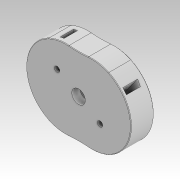
# Autodesk Inventor part: Rotor_NEW
Saved by Autodesk Inventor 2020 (Build 240168000, 168)
## iProperties
Created: 2022-01-30
Part Number: Rotor_NEW
Material: Generic
Document SubType Name: Modeling
Designer: DDeGo
Density: 1 g/cm^3
Appearance: Default
Author: DDeGo
Autodesk Inventor part; units mm, degrees
ref_plane "YZ Plane" through (0, 0, 0) normal (1, 0, 0) x (0, 1, 0)
ref_plane "XZ Plane" through (0, 0, 0) normal (0, 1, 0) x (-1, 0, 0)
ref_plane "XY Plane" through (0, 0, 0) normal (0, 0, 1) x (1, 0, 0)
sketch "Sketch1" plane through (0, 0, 0) normal (0, 0, 1) x (1, 0, 0)
  line L0 (4.8, 0) -> (-4.8, 0) construction
  line L1 (4.8, 14.7) -> (-4.8, 14.7) construction
  arc A0 (19.5, 0) -> (11.1318, 13.2664) centre (4.8, 0) ccw
  arc A1 (-4.8, 14.7) -> (-11.1318, 13.2664) centre (-4.8, 0) ccw construction
  line L2 (-19.5, 24.8831) -> (19.5, 24.8831) construction
  line L3 (19.5, 24.8831) -> (19.5, -24.8831) construction
  line L4 (19.5, -24.8831) -> (-19.5, -24.8831) construction
  line L5 (-19.5, -24.8831) -> (-19.5, 24.8831) construction
  line L6 (0, 0) -> (0, 14.7) construction
  arc A2 (-3.6434, 14.6131) -> (0, 14.45) centre (0, 55.2356) ccw
  arc A3 (-3.6434, 14.6131) -> (-11.1318, 13.2664) centre (-4.9297, 0.2718) ccw
  arc A4 (-11.1318, 13.2664) -> (-19.5, 0) centre (-4.8, 0) ccw
  arc A5 (0, 14.45) -> (3.6434, 14.6131) centre (0, 55.2356) ccw
  arc A6 (11.1318, 13.2664) -> (3.6434, 14.6131) centre (4.9297, 0.2718) ccw
  arc A7 (11.1318, 13.2664) -> (4.8, 14.7) centre (4.8, 0) ccw construction
  line L7 (-19.5, 0) -> (19.5, 0) construction
  arc A8 (11.1318, -13.2664) -> (19.5, 0) centre (4.8, 0) ccw
  arc A9 (0, -14.45) -> (-3.6434, -14.6131) centre (0, -55.2356) ccw
  arc A10 (-11.1318, -13.2664) -> (-3.6434, -14.6131) centre (-4.9297, -0.2718) ccw
  arc A11 (-19.5, 0) -> (-11.1318, -13.2664) centre (-4.8, 0) ccw
  arc A12 (3.6434, -14.6131) -> (0, -14.45) centre (0, -55.2356) ccw
  arc A13 (3.6434, -14.6131) -> (11.1318, -13.2664) centre (4.9297, -0.2718) ccw
  circle A14 centre (0, 0) radius 2.5
  line L8 (-11.1318, 13.2664) -> (0, 0) construction
  line L9 (-3.6434, 14.6131) -> (0, 0) construction
  dimension "d0" = 14.7
  dimension "d1" = 39
  dimension "d2" = 0.25
  dimension "d5" = 5
  dimension "d14" = 40
  dimension "d15" = 14
  constraints: 28 point on circle, 22 end point, 15 centre point, 12 tangent, 9 symmetric about line, 5 midpoint, 3 point on line, 2 equal radius, 2 horizontal, 2 parallel, 1 coincident, 1 perpendicular, 1 vertical, 6 other
  measures "d0" radius of A1
  measures "d1" distance of L2.start L2.end
  measures "d2" distance from line of L1 A2.end
  measures "d5" diameter of A14
  measures "d14" angle of L6 L8
  measures "d15" angle of L6 L9
extrude "Extrusion1" add sketch "Sketch1" along normal mid plane 8 contours A8 A13 A12 A9 A10 A11 A4 A3 A2 A5 A6 A0 | A14
sketch "Sketch2" plane through (0, 0, 0) normal (0, 1, 0) x (-1, 0, 0)
  line L0 (0, 0) -> (0, 4) construction
  line L1 (0, 4) -> (2.52, 4)
  line L2 (-3.6434, 4) -> (3.6434, 4) construction
  line L3 (3.6434, 4) -> (11.1318, 4) construction
  line L4 (11.1318, 4) -> (11.1318, 4) construction
  line L5 (11.1318, 4) -> (3.6434, 4) construction
  line L6 (3.6434, 4) -> (-3.6434, 4) construction
  line L7 (-3.6434, 4) -> (-11.1318, 4) construction
  line L8 (-11.1318, 4) -> (-11.1318, 4) construction
  line L9 (-11.1318, 4) -> (-3.6434, 4) construction
  line L10 (2.52, -4) -> (0, -4)
  line L11 (0, -4) -> (0, 4)
  line L12 (3.6434, -4) -> (-3.6434, -4) projected
  line L13 (-3.6434, -4) -> (-11.1318, -4) projected
  line L14 (-11.1318, -4) -> (-11.1318, -4) projected
  line L15 (-11.1318, -4) -> (-3.6434, -4) projected
  line L16 (-3.6434, -4) -> (3.6434, -4) projected
  line L17 (3.6434, -4) -> (11.1318, -4) projected
  line L18 (11.1318, -4) -> (11.1318, -4) projected
  line L19 (11.1318, -4) -> (3.6434, -4) projected
  line L20 (2.52, -1) -> (2.02, -0.7113)
  line L21 (2.02, -0.7113) -> (2.02, 0.7113)
  line L22 (2.02, 0.7113) -> (2.52, 1)
  line L23 (2.52, 4) -> (2.52, 1)
  line L24 (2.52, -1) -> (2.52, -4)
  dimension "d53" = 2.52
  dimension "d54" = 0.5
  dimension "d55" = 60
  dimension "d56" = 3
  dimension "d57" = 3
  constraints: 18 end point, 2 collinear, 2 midpoint, 2 perpendicular, 2 vertical, 1 equal length, 1 horizontal, 1 point on line
  measures "d53" distance between parallel lines of L24 L11
  measures "d54" distance between parallel lines of L24 L21
  measures "d55" angle of L24 L20
  measures "d56" distance of L1.end L22.end
  measures "d57" distance of L20.start L10.start
revolve "Revolution1" cut sketch "Sketch2" angle 360 about axis through (0, 0, 0) along (0, 0, 1)
sketch "Sketch3" plane through (0, 0, -4) normal (0, 0, -1) x (-1, 0, 0)
  circle A0 centre (0, 0) radius 12.5
  circle A1 centre (0, 0) radius 2.5 projected
  dimension "d18" = 25
  constraints: 1 centre point, 1 coincident
  measures "d18" diameter of A0
extrude "Extrusion2" add sketch "Sketch3" along normal blind 10
spur gear teeth "Spur Gear1" teeth 16 pitch diameter 9.6 tip diameter 10.6669 root diameter 7.9669 face width 3 trims to tip circle yes start plane through (0, 0, -14) normal (0, 0, -1) x (-1, 0, 0)
ref_plane "Work Plane1" through (0, 0, -0.5) normal (0, 0, -1) x (-1, 0, 0)
sketch "Sketch4" plane through (0, 0, -11) normal (0, 0, -1) x (-1, 0, 0)
  arc A0 (3.9518, 3.5817) -> (3.5817, 3.9518) centre (0, 0) ccw projected
  arc A1 (3.1996, 2.3729) -> (3.9518, 3.5817) centre (-0.1257, 5.2809) ccw projected
  arc A2 (4.8214, 2.2804) -> (3.4167, 2.0479) centre (4.8308, -2.137) ccw projected
  arc A3 (5.0217, 1.7968) -> (4.8214, 2.2804) centre (0, 0) ccw projected
  arc A4 (3.8641, 0.9679) -> (5.0217, 1.7968) centre (1.9048, 4.927) ccw projected
  arc A5 (5.327, 0.2617) -> (3.9404, 0.5845) centre (3.6453, -3.823) ccw projected
  arc A6 (5.327, -0.2617) -> (5.327, 0.2617) centre (0, 0) ccw projected
  arc A7 (3.9404, -0.5845) -> (5.327, -0.2617) centre (3.6453, 3.823) ccw projected
  arc A8 (5.0217, -1.7968) -> (3.8641, -0.9679) centre (1.9048, -4.927) ccw projected
  arc A9 (4.8214, -2.2804) -> (5.0217, -1.7968) centre (0, 0) ccw projected
  arc A10 (3.4167, -2.0479) -> (4.8214, -2.2804) centre (4.8308, 2.137) ccw projected
  arc A11 (3.9518, -3.5817) -> (3.1996, -2.3729) centre (-0.1257, -5.2809) ccw projected
  arc A12 (3.5817, -3.9518) -> (3.9518, -3.5817) centre (0, 0) ccw projected
  arc A13 (2.3729, -3.1996) -> (3.5817, -3.9518) centre (5.2809, 0.1257) ccw projected
  arc A14 (2.2804, -4.8214) -> (2.0479, -3.4167) centre (-2.137, -4.8308) ccw projected
  arc A15 (1.7968, -5.0217) -> (2.2804, -4.8214) centre (0, 0) ccw projected
  arc A16 (0.9679, -3.8641) -> (1.7968, -5.0217) centre (4.927, -1.9048) ccw projected
  arc A17 (0.2617, -5.327) -> (0.5845, -3.9404) centre (-3.823, -3.6453) ccw projected
  arc A18 (-0.2617, -5.327) -> (0.2617, -5.327) centre (0, 0) ccw projected
  arc A19 (-0.5845, -3.9404) -> (-0.2617, -5.327) centre (3.823, -3.6453) ccw projected
  arc A20 (-1.7968, -5.0217) -> (-0.9679, -3.8641) centre (-4.927, -1.9048) ccw projected
  arc A21 (-2.2804, -4.8214) -> (-1.7968, -5.0217) centre (0, 0) ccw projected
  arc A22 (-2.0479, -3.4167) -> (-2.2804, -4.8214) centre (2.137, -4.8308) ccw projected
  arc A23 (-3.5817, -3.9518) -> (-2.3729, -3.1996) centre (-5.2809, 0.1257) ccw projected
  arc A24 (-3.9518, -3.5817) -> (-3.5817, -3.9518) centre (0, 0) ccw projected
  arc A25 (-3.1996, -2.3729) -> (-3.9518, -3.5817) centre (0.1257, -5.2809) ccw projected
  arc A26 (-4.8214, -2.2804) -> (-3.4167, -2.0479) centre (-4.8308, 2.137) ccw projected
  arc A27 (-5.0217, -1.7968) -> (-4.8214, -2.2804) centre (0, 0) ccw projected
  arc A28 (-3.8641, -0.9679) -> (-5.0217, -1.7968) centre (-1.9048, -4.927) ccw projected
  arc A29 (-5.327, -0.2617) -> (-3.9404, -0.5845) centre (-3.6453, 3.823) ccw projected
  arc A30 (-5.327, 0.2617) -> (-5.327, -0.2617) centre (0, 0) ccw projected
  arc A31 (-3.9404, 0.5845) -> (-5.327, 0.2617) centre (-3.6453, -3.823) ccw projected
  arc A32 (-5.0217, 1.7968) -> (-3.8641, 0.9679) centre (-1.9048, 4.927) ccw projected
  arc A33 (-4.8214, 2.2804) -> (-5.0217, 1.7968) centre (0, 0) ccw projected
  arc A34 (-3.4167, 2.0479) -> (-4.8214, 2.2804) centre (-4.8308, -2.137) ccw projected
  arc A35 (-3.9518, 3.5817) -> (-3.1996, 2.3729) centre (0.1257, 5.2809) ccw projected
  arc A36 (-3.5817, 3.9518) -> (-3.9518, 3.5817) centre (0, 0) ccw projected
  arc A37 (-2.3729, 3.1996) -> (-3.5817, 3.9518) centre (-5.2809, -0.1257) ccw projected
  arc A38 (-2.2804, 4.8214) -> (-2.0479, 3.4167) centre (2.137, 4.8308) ccw projected
  arc A39 (-1.7968, 5.0217) -> (-2.2804, 4.8214) centre (0, 0) ccw projected
  arc A40 (-0.9679, 3.8641) -> (-1.7968, 5.0217) centre (-4.927, 1.9048) ccw projected
  arc A41 (-0.2617, 5.327) -> (-0.5845, 3.9404) centre (3.823, 3.6453) ccw projected
  arc A42 (0.2617, 5.327) -> (-0.2617, 5.327) centre (0, 0) ccw projected
  arc A43 (0.5845, 3.9404) -> (0.2617, 5.327) centre (-3.823, 3.6453) ccw projected
  arc A44 (1.7968, 5.0217) -> (0.9679, 3.8641) centre (4.927, 1.9048) ccw projected
  arc A45 (2.2804, 4.8214) -> (1.7968, 5.0217) centre (0, 0) ccw projected
  arc A46 (2.0479, 3.4167) -> (2.2804, 4.8214) centre (-2.137, 4.8308) ccw projected
  arc A47 (3.5817, 3.9518) -> (2.3729, 3.1996) centre (5.2809, -0.1257) ccw projected
  circle A48 centre (0, 0) radius 12.5 projected
  arc A49 (3.4167, 2.0479) -> (3.1996, 2.3729) centre (0, 0) ccw projected
  arc A50 (3.9404, 0.5845) -> (3.8641, 0.9679) centre (0, 0) ccw projected
  arc A51 (3.8641, -0.9679) -> (3.9404, -0.5845) centre (0, 0) ccw projected
  arc A52 (3.1996, -2.3729) -> (3.4167, -2.0479) centre (0, 0) ccw projected
  arc A53 (2.0479, -3.4167) -> (2.3729, -3.1996) centre (0, 0) ccw projected
  arc A54 (0.5845, -3.9404) -> (0.9679, -3.8641) centre (0, 0) ccw projected
  arc A55 (-0.9679, -3.8641) -> (-0.5845, -3.9404) centre (0, 0) ccw projected
  arc A56 (-2.3729, -3.1996) -> (-2.0479, -3.4167) centre (0, 0) ccw projected
  arc A57 (-3.4167, -2.0479) -> (-3.1996, -2.3729) centre (0, 0) ccw projected
  arc A58 (-3.9404, -0.5845) -> (-3.8641, -0.9679) centre (0, 0) ccw projected
  arc A59 (-3.8641, 0.9679) -> (-3.9404, 0.5845) centre (0, 0) ccw projected
  arc A60 (-3.1996, 2.3729) -> (-3.4167, 2.0479) centre (0, 0) ccw projected
  arc A61 (-2.0479, 3.4167) -> (-2.3729, 3.1996) centre (0, 0) ccw projected
  arc A62 (-0.5845, 3.9404) -> (-0.9679, 3.8641) centre (0, 0) ccw projected
  arc A63 (0.9679, 3.8641) -> (0.5845, 3.9404) centre (0, 0) ccw projected
  arc A64 (2.3729, 3.1996) -> (2.0479, 3.4167) centre (0, 0) ccw projected
  point P0 (0, 0)
extrude "Extrusion3" cut sketch "Sketch4" against normal up to surface (10.5 mm away)
ref_plane "Work Plane2" through (0, 0, -3.75) normal (0, 0, -1) x (-1, 0, 0)
sketch "Sketch5" plane through (0, 0, -14) normal (0, 0, -1) x (-1, 0, 0)
  circle A0 centre (0, 0) radius 7.9397
  constraints: 1 centre point, 1 coincident
extrude "Extrusion4" cut sketch "Sketch5" against normal up to surface (10.25 mm away)
fillet "Fillet1" radius 0.3 32 edges at (-1.7968, -5.0217, -2.125) (-2.2804, -4.8214, -2.125) (-3.5817, -3.9518, -2.125) (-3.9518, -3.5817, -2.125) (-5.0217, -1.7968, -2.125) (-4.8214, -2.2804, -2.125) (-5.327, -0.2617, -2.125) (-5.327, 0.2617, -2.125) (-5.0217, 1.7968, -2.125) (-4.8214, 2.2804, -2.125) (-3.9518, 3.5817, -2.125) (-3.5817, 3.9518, -2.125) (-2.2804, 4.8214, -2.125) (-1.7968, 5.0217, -2.125) (-0.2617, 5.327, -2.125) (0.2617, 5.327, -2.125) (2.2804, 4.8214, -2.125) (1.7968, 5.0217, -2.125) (3.5817, 3.9518, -2.125) (3.9518, 3.5817, -2.125) (4.8214, 2.2804, -2.125) (5.0217, 1.7968, -2.125) (5.327, 0.2617, -2.125) (5.327, -0.2617, -2.125) (5.0217, -1.7968, -2.125) (4.8214, -2.2804, -2.125) (3.9518, -3.5817, -2.125) (3.5817, -3.9518, -2.125) (2.2804, -4.8214, -2.125) (1.7968, -5.0217, -2.125) (0.2617, -5.327, -2.125) (-0.2617, -5.327, -2.125)
fillet "Fillet2" radius 1 1 edges at (12.5, 0, -0.5)
sketch "Sketch6" plane through (0, 0, 4) normal (0, 0, 1) x (1, 0, 0)
  circle A0 centre (8, -4.8) radius 1
  circle A1 centre (9.6805, -3.2071) radius 1.1297 construction
  line L0 (0, 0) -> (8, -4.8) construction
  line L1 (8, -4.8) -> (8, 0) construction
  line L2 (8, 0) -> (0, 0) construction
  dimension "d28" = 8
  dimension "d29" = 4.8
  dimension "d30" = 2
  constraints: 6 end point, 2 centre point, 1 perpendicular, 1 vertical
  measures "d28" distance of L1.end L0.start
  measures "d29" distance of L0.end L1.end
  measures "d30" diameter of A0
extrude "Extrusion5" cut sketch "Sketch6" against normal blind 3.5
sketch "Sketch7" plane through (8, -4.8, 0.5) normal (0, 0, 1) x (1, 0, 0)
  circle A0 centre (0, 0) radius 1 construction
  line L0 (0, 0) -> (10.4256, 18.0576) construction
  line L1 (-0.866, 0.5) -> (9.5595, 18.5576)
  line L2 (11.2916, 17.5576) -> (0.866, -0.5)
  arc A1 (-0.866, 0.5) -> (0.866, -0.5) centre (0, 0) ccw
  arc A2 (11.2916, 17.5576) -> (9.5595, 18.5576) centre (10.4256, 18.0576) ccw
  circle A3 centre (0, 0) radius 1 projected
  line L3 (0, 0) -> (0, 4.6154) construction
  point P0 (-8, 4.8)
  point P1 (5.2128, 9.0288)
  point P2 (-0.866, 0.5)
  point P3 (0.866, -0.5)
  dimension "d33" = 30
  constraints: 10 end point, 4 point on circle, 4 tangent, 2 centre point, 1 concentric, 1 midpoint, 1 parallel, 1 vertical
  measures "d33" angle of L0 L3
extrude "Extrusion6" cut sketch "Sketch7" along normal blind 2.5 contours L1 A2 L2 A3
sketch "Sketch8" plane through (15.4603, 10.1216, 3) normal (0.8660254, -0.5, 0) x (0, 0, -1)
  line L0 (0, 0) -> (2.5, 0) construction
  line L1 (0, 0) -> (0, -16.6527) construction
  line L2 (2.5, -16.6527) -> (0, -16.6527) construction
  line L3 (2.5, 0) -> (2.5, -16.6527) construction
  line L4 (2.5, 0) -> (2.5, -16.6527) construction
  line L5 (2.5, -7.6527) -> (5.5, 0)
  line L6 (5.5, 0) -> (2.5, 0)
  line L7 (7, 0.5592) -> (-1, 0.5592) construction
  line L8 (2.5, 0) -> (2.5, -7.6527)
  line L9 (7, -22.4189) -> (7, 0.6042) construction
  point P0 (3, -16.4958)
  dimension "d36" = 9
  dimension "d38" = 1.5
  constraints: 6 end point, 1 parallel, 1 perpendicular, 1 point on line
  measures "d36" distance from line of L5.start L2
  measures "d38" distance from line of L9 L5.end
extrude "Extrusion7" cut sketch "Sketch8" along normal up to surface (2 mm away)
sketch "Sketch9" plane through (0, 0, 0) normal (0, 0, 1) x (1, 0, 0)
  line L0 (7.1255, -15.5449) -> (6.7355, -13.5833)
  line L1 (6.7355, -13.5833) -> (8.2068, -13.2908)
  line L2 (8.2068, -13.2908) -> (8.5967, -15.2525)
  line L3 (8.5967, -15.2525) -> (7.1255, -15.5449)
  line L4 (7.1255, -15.5449) -> (8.2068, -13.2908) construction
  line L5 (6.7355, -13.5833) -> (8.5967, -15.2525) construction
  arc A0 (11.1318, -13.2664) -> (11.1318, 13.2664) centre (4.8, 0) ccw projected
  arc A1 (3.6434, -14.6131) -> (11.1318, -13.2664) centre (4.9297, -0.2718) ccw projected
  line L6 (7.6661, -14.4179) -> (7.4711, -13.4371)
  line L7 (0, 0) -> (7.6661, -14.4179) construction
  circle A2 centre (0, 0) radius 2.02 projected
  line L8 (0, 0) -> (0, -15.7126) construction
  dimension "d43" = 1.5
  dimension "d44" = 2
  dimension "d58" = 28
  constraints: 18 end point, 4 midpoint, 2 parallel, 1 line through centre, 1 perpendicular, 1 point on circle, 1 vertical
  measures "d43" distance between parallel lines of L0 L2
  measures "d44" distance between parallel lines of L3 L1
  measures "d58" angle of L7 L8
extrude "Extrusion8" cut sketch "Sketch9" against normal mid plane 5 contours L0 A1 L2 L3 | L0 L1 L6 A1 | L6 L1 L2 A1
sketch "Sketch10" plane through (8.3798, -14.1615, -2.5) normal (-0.9808083, -0.1949744, 0) x (0, 0, 1)
  line L0 (5, -0.0871) -> (5, 0.8877) projected
  line L1 (0, 0.8877) -> (5, 0.8877) projected
  line L2 (0, 0.8877) -> (0, -0.0871) projected
  line L3 (0, 0.8877) -> (5, 0.8877) projected
  line L4 (5, 0.8877) -> (1, 7.0236)
  line L5 (1, 7.0236) -> (-1.5, 7.0236)
  line L6 (-1.5, 7.0236) -> (0, 0.8877)
  line L7 (-1.5, 3.0236) -> (-1.5, 28.0236) construction
  line L8 (-1.5, 30.5666) -> (-1.5, 29.1458) projected
  line L9 (-1.5, 29.1458) -> (-1.5, 26.365) projected
  line L10 (-1.5, 26.365) -> (-1.5, 0.3414) construction
  line L11 (-1.5, 0.3414) -> (-1.5, 0.4806) construction
  line L12 (-1.5, 0.4806) -> (-1.5, 1.9014) construction
  line L13 (-1.5, 1.9014) -> (-1.5, 4.6822) construction
  line L14 (-1.5, 4.6822) -> (-1.5, 30.7058) construction
  line L15 (-1.5, 30.7058) -> (-1.5, 30.5666) projected
  line L16 (-1.5, 3.0236) -> (-1.5, 28.0236) construction
  line L17 (1, 28.0236) -> (1, 3.0236) construction
  line L18 (-1.5, 3.0236) -> (1, 3.0236) construction
  line L19 (5, -0.0871) -> (0, -0.0871) projected
  point P0 (2.5, 15.5236)
  dimension "d45" = 4
  constraints: 6 end point, 2 point on line, 1 parallel
  measures "d45" distance from line of L18 L5.end
extrude "Extrusion9" cut sketch "Sketch10" along normal up to surface (1.5 mm away) contours L1 L6 L5 L4
fillet "Fillet3" radius 2 6 edges at (6.1937, -10.8576, -2.3397) (5.9127, -9.4441, -0.5) (6.1323, -10.5485, -0.7873) (7.3181, -8.8206, -0.5) (7.5457, -9.9655, -2.4144) (7.4795, -9.6324, -0.7813)
pattern_circular "Circular Pattern1" count 2 over 360 about axis through (0, 0, -2.5) along (0, 0, -1) of "Extrusion5", "Extrusion6", "Extrusion7", "Extrusion8", "Extrusion9", "Fillet3"
sketch "Sketch12" plane through (0, 0, -4) normal (0, 0, -1) x (-1, 0, 0)
  circle A0 centre (0, 0) radius 12.5 projected
  arc A1 (-3.6434, 14.6131) -> (3.6434, 14.6131) centre (0, 55.2356) ccw projected
  arc A2 (-3.6434, 14.6131) -> (-11.1318, 13.2664) centre (-4.9297, 0.2718) ccw projected
  arc A3 (-11.1318, 13.2664) -> (-11.1318, -13.2664) centre (-4.8, 0) ccw projected
  arc A4 (-11.1318, -13.2664) -> (-3.6434, -14.6131) centre (-4.9297, -0.2718) ccw projected
  arc A5 (3.6434, -14.6131) -> (-3.6434, -14.6131) centre (0, -55.2356) ccw projected
  arc A6 (3.6434, -14.6131) -> (11.1318, -13.2664) centre (4.9297, -0.2718) ccw projected
  arc A7 (11.1318, -13.2664) -> (11.1318, 13.2664) centre (4.8, 0) ccw projected
  arc A8 (11.1318, 13.2664) -> (3.6434, 14.6131) centre (4.9297, 0.2718) ccw projected
  arc A9 (3.7328, -13.6171) -> (10.7011, -12.3639) centre (4.9297, -0.2718) ccw
  arc A10 (3.7328, -13.6171) -> (-3.7328, -13.6171) centre (0, -55.2356) ccw
  arc A11 (-10.7011, -12.3639) -> (-3.7328, -13.6171) centre (-4.9297, -0.2718) ccw
  arc A12 (-10.7011, 12.3639) -> (-10.7011, -12.3639) centre (-4.8, 0) ccw
  arc A13 (-3.7328, 13.6171) -> (-10.7011, 12.3639) centre (-4.9297, 0.2718) ccw
  arc A14 (-3.7328, 13.6171) -> (3.7328, 13.6171) centre (0, 55.2356) ccw
  arc A15 (10.7011, 12.3639) -> (3.7328, 13.6171) centre (4.9297, 0.2718) ccw
  arc A16 (10.7011, -12.3639) -> (10.7011, 12.3639) centre (4.8, 0) ccw
  dimension "d0" = 14.7
  dimension "d1" = 39
  dimension "d2" = 0.25
  dimension "d5" = 5
  dimension "d14" = 40
  dimension "d15" = 14
  dimension "d60" = 1
  constraints: 16 point on circle, 8 centre point, 7 other
  measures "d60" radial gap between concentric circles of A6 A9
extrude "Extrusion10" add sketch "Sketch12" along normal blind 0.5 contours A1 A8 A7 A6 A5 A4 A3 A2
fillet "Fillet4" radius 10 1 edges at (12.5, 2.9942, 0.5)
sketch "Sketch13" plane through (3.823, -3.6453, -3.75) normal (0, 0, -1) x (-0.9789933, -0.2038926, 0)
  arc A0 (4.1422, -0.8614) -> (4.3751, -0.6098) centre (4.0779, -0.5684) ccw projected
  arc A1 (4.3751, -0.6098) -> (4.3751, 0.6098) centre (0, 0) ccw projected
  arc A2 (4.3751, 0.6098) -> (4.7349, 0.7626) centre (2.9994, 4.3482) ccw projected
  arc A3 (4.7349, 0.7626) -> (5.6126, -0.0841) centre (8.2113, 3.488) ccw projected
  arc A4 (5.6126, -0.0841) -> (5.9554, -0.0912) centre (5.7891, 0.1585) ccw projected
  arc A5 (5.9554, -0.0912) -> (6.0489, -0.0275) centre (2.9994, 4.3482) ccw projected
  arc A6 (6.0489, -0.0275) -> (6.1677, 0.294) centre (5.8773, 0.2186) ccw projected
  arc A7 (6.1677, 0.294) -> (5.701, 1.4208) centre (1.8923, -0.8169) ccw projected
  arc A8 (5.701, 1.4208) -> (5.9749, 1.6997) centre (2.9994, 4.3482) ccw projected
  arc A9 (5.9749, 1.6997) -> (7.1099, 1.2533) centre (8.1438, 5.5479) ccw projected
  arc A10 (7.1099, 1.2533) -> (7.4292, 1.3779) centre (7.1801, 1.545) ccw projected
  arc A11 (7.4292, 1.3779) -> (7.4913, 1.4725) centre (2.9994, 4.3482) ccw projected
  arc A12 (7.4913, 1.4725) -> (7.478, 1.8151) centre (7.2386, 1.6343) ccw projected
  arc A13 (7.478, 1.8151) -> (6.6156, 2.6775) centre (3.9532, -0.8474) ccw projected
  arc A14 (6.6156, 2.6775) -> (6.762, 3.0399) centre (2.9994, 4.3482) ccw projected
  arc A15 (6.762, 3.0399) -> (7.9813, 3.0619) centre (7.2931, 7.4253) ccw projected
  arc A16 (7.9813, 3.0619) -> (8.2287, 3.2992) centre (7.9346, 3.3582) ccw projected
  arc A17 (8.2287, 3.2992) -> (8.2498, 3.4104) centre (2.9994, 4.3482) ccw projected
  arc A18 (8.2498, 3.4104) -> (8.1065, 3.7218) centre (7.9545, 3.4631) ccw projected
  arc A19 (8.1065, 3.7218) -> (6.9797, 4.1885) centre (5.8688, -0.0869) ccw projected
  arc A20 (6.9797, 4.1885) -> (6.9762, 4.5794) centre (2.9994, 4.3482) ccw projected
  arc A21 (6.9762, 4.5794) -> (8.0944, 5.0663) centre (5.7887, 8.8341) ccw projected
  arc A22 (8.0944, 5.0663) -> (8.2321, 5.3802) centre (7.9378, 5.3222) ccw projected
  arc A23 (8.2321, 5.3802) -> (8.209, 5.491) centre (2.9994, 4.3482) ccw projected
  arc A24 (8.209, 5.491) -> (7.9574, 5.7238) centre (7.916, 5.4267) ccw projected
  arc A25 (7.9574, 5.7238) -> (6.7378, 5.7238) centre (7.3476, 1.3487) ccw projected
  arc A26 (6.7378, 5.7238) -> (6.585, 6.0836) centre (2.9994, 4.3482) ccw projected
  arc A27 (6.585, 6.0836) -> (7.4318, 6.9613) centre (3.8597, 9.5601) ccw projected
  arc A28 (7.4318, 6.9613) -> (7.4389, 7.3041) centre (7.1892, 7.1378) ccw projected
  arc A29 (7.4389, 7.3041) -> (7.3752, 7.3976) centre (2.9994, 4.3482) ccw projected
  arc A30 (7.3752, 7.3976) -> (7.0536, 7.5164) centre (7.129, 7.2261) ccw projected
  arc A31 (7.0536, 7.5164) -> (5.9269, 7.0497) centre (8.1645, 3.241) ccw projected
  arc A32 (5.9269, 7.0497) -> (5.648, 7.3237) centre (2.9994, 4.3482) ccw projected
  arc A33 (5.648, 7.3237) -> (6.0944, 8.4586) centre (1.7997, 9.4925) ccw projected
  arc A34 (6.0944, 8.4586) -> (5.9698, 8.778) centre (5.8027, 8.5288) ccw projected
  arc A35 (5.9698, 8.778) -> (5.8751, 8.84) centre (2.9994, 4.3482) ccw projected
  arc A36 (5.8751, 8.84) -> (5.5326, 8.8267) centre (5.7134, 8.5873) ccw projected
  arc A37 (5.5326, 8.8267) -> (4.6702, 7.9644) centre (8.195, 5.3019) ccw projected
  arc A38 (4.6702, 7.9644) -> (4.3077, 8.1107) centre (2.9994, 4.3482) ccw projected
  arc A39 (4.3077, 8.1107) -> (4.2858, 9.3301) centre (-0.0776, 8.6418) ccw projected
  arc A40 (4.2858, 9.3301) -> (4.0484, 9.5775) centre (3.9894, 9.2833) ccw projected
  arc A41 (4.0484, 9.5775) -> (3.9373, 9.5986) centre (2.9994, 4.3482) ccw projected
  arc A42 (3.9373, 9.5986) -> (3.6259, 9.4552) centre (3.8845, 9.3032) ccw projected
  arc A43 (3.6259, 9.4552) -> (3.1592, 8.3285) centre (7.4346, 7.2176) ccw projected
  arc A44 (3.1592, 8.3285) -> (2.7683, 8.3249) centre (2.9994, 4.3482) ccw projected
  arc A45 (2.7683, 8.3249) -> (2.2814, 9.4431) centre (-1.4865, 7.1374) ccw projected
  arc A46 (2.2814, 9.4431) -> (1.9674, 9.5809) centre (2.0255, 9.2865) ccw projected
  arc A47 (1.9674, 9.5809) -> (1.8567, 9.5578) centre (2.9994, 4.3482) ccw projected
  arc A48 (1.8567, 9.5578) -> (1.6238, 9.3062) centre (1.9209, 9.2648) ccw projected
  arc A49 (1.6238, 9.3062) -> (1.6238, 8.0866) centre (5.9989, 8.6964) ccw projected
  arc A50 (1.6238, 8.0866) -> (1.264, 7.9338) centre (2.9994, 4.3482) ccw projected
  arc A51 (1.264, 7.9338) -> (0.3863, 8.7805) centre (-2.2124, 5.2084) ccw projected
  arc A52 (0.3863, 8.7805) -> (0.0435, 8.7876) centre (0.2098, 8.5379) ccw projected
  arc A53 (0.0435, 8.7876) -> (-0.05, 8.7239) centre (2.9994, 4.3482) ccw projected
  arc A54 (-0.05, 8.7239) -> (-0.1688, 8.4023) centre (0.1216, 8.4778) ccw projected
  arc A55 (-0.1688, 8.4023) -> (0.2979, 7.2756) centre (4.1066, 9.5132) ccw projected
  arc A56 (0.2979, 7.2756) -> (0.024, 6.9967) centre (2.9994, 4.3482) ccw projected
  arc A57 (0.024, 6.9967) -> (-1.111, 7.4431) centre (-2.1449, 3.1484) ccw projected
  arc A58 (-1.111, 7.4431) -> (-1.4304, 7.3185) centre (-1.1812, 7.1514) ccw projected
  arc A59 (-1.4304, 7.3185) -> (-1.4924, 7.2239) centre (2.9994, 4.3482) ccw projected
  arc A60 (-1.4924, 7.2239) -> (-1.4791, 6.8813) centre (-1.2397, 7.0621) ccw projected
  arc A61 (-1.4791, 6.8813) -> (-0.6167, 6.0189) centre (2.0457, 9.5438) ccw projected
  arc A62 (-0.6167, 6.0189) -> (-0.7631, 5.6564) centre (2.9994, 4.3482) ccw projected
  arc A63 (-0.7631, 5.6564) -> (-1.9824, 5.6345) centre (-1.2942, 1.2711) ccw projected
  arc A64 (-1.9824, 5.6345) -> (-2.2298, 5.3972) centre (-1.9357, 5.3382) ccw projected
  arc A65 (-2.2298, 5.3972) -> (-2.2509, 5.286) centre (2.9994, 4.3482) ccw projected
  arc A66 (-2.2509, 5.286) -> (-2.1076, 4.9746) centre (-1.9556, 5.2333) ccw projected
  arc A67 (-2.1076, 4.9746) -> (-0.9808, 4.5079) centre (0.1301, 8.7833) ccw projected
  arc A68 (-0.9808, 4.5079) -> (-0.9773, 4.117) centre (2.9994, 4.3482) ccw projected
  arc A69 (-0.9773, 4.117) -> (-2.0955, 3.6301) centre (0.2102, -0.1377) ccw projected
  arc A70 (-2.0955, 3.6301) -> (-2.2332, 3.3162) centre (-1.9389, 3.3742) ccw projected
  arc A71 (-2.2332, 3.3162) -> (-2.2102, 3.2054) centre (2.9994, 4.3482) ccw projected
  arc A72 (-2.2102, 3.2054) -> (-1.9585, 2.9726) centre (-1.9171, 3.2697) ccw projected
  arc A73 (-1.9585, 2.9726) -> (-0.739, 2.9726) centre (-1.3487, 7.3476) ccw projected
  arc A74 (-0.739, 2.9726) -> (-0.5861, 2.6128) centre (2.9994, 4.3482) ccw projected
  arc A75 (-0.5861, 2.6128) -> (-1.4329, 1.735) centre (2.1392, -0.8637) ccw projected
  arc A76 (-1.4329, 1.735) -> (-1.44, 1.3923) centre (-1.1903, 1.5586) ccw projected
  arc A77 (-1.44, 1.3923) -> (-1.3763, 1.2988) centre (2.9994, 4.3482) ccw projected
  arc A78 (-1.3763, 1.2988) -> (-1.0547, 1.1799) centre (-1.1301, 1.4703) ccw projected
  arc A79 (-1.0547, 1.1799) -> (0.072, 1.6467) centre (-2.1656, 5.4553) ccw projected
  arc A80 (0.072, 1.6467) -> (0.3509, 1.3727) centre (2.9994, 4.3482) ccw projected
  arc A81 (0.3509, 1.3727) -> (-0.0955, 0.2378) centre (4.1992, -0.7961) ccw projected
  arc A82 (-0.0955, 0.2378) -> (0.0291, -0.0816) centre (0.1962, 0.1676) ccw projected
  arc A83 (0.0291, -0.0816) -> (0.1238, -0.1436) centre (2.9994, 4.3482) ccw projected
  arc A84 (0.1238, -0.1436) -> (0.4663, -0.1303) centre (0.2855, 0.109) ccw projected
  arc A85 (0.4663, -0.1303) -> (1.3287, 0.732) centre (-2.1961, 3.3945) ccw projected
  arc A86 (1.3287, 0.732) -> (1.6912, 0.5857) centre (2.9994, 4.3482) ccw projected
  arc A87 (1.6912, 0.5857) -> (1.7131, -0.6337) centre (6.0765, 0.0546) ccw projected
  arc A88 (1.7131, -0.6337) -> (1.9504, -0.8811) centre (2.0094, -0.587) ccw projected
  arc A89 (1.9504, -0.8811) -> (2.0616, -0.9022) centre (2.9994, 4.3482) ccw projected
  arc A90 (2.0616, -0.9022) -> (2.373, -0.7588) centre (2.1144, -0.6068) ccw projected
  arc A91 (2.373, -0.7588) -> (2.8397, 0.3679) centre (-1.4357, 1.4788) ccw projected
  arc A92 (2.8397, 0.3679) -> (3.2306, 0.3714) centre (2.9994, 4.3482) ccw projected
  arc A93 (3.2306, 0.3714) -> (3.7175, -0.7467) centre (7.4854, 1.559) ccw projected
  arc A94 (3.7175, -0.7467) -> (4.0315, -0.8845) centre (3.9734, -0.5901) ccw projected
  arc A95 (4.0315, -0.8845) -> (4.1422, -0.8614) centre (2.9994, 4.3482) ccw projected
  circle A96 centre (2.9994, 4.3482) radius 2.52 projected
  arc A97 (4.7494, 0.8254) -> (5.642, -0.0437) centre (8.2113, 3.488) ccw
  arc A98 (4.3198, 0.6429) -> (4.7494, 0.8254) centre (2.9994, 4.3482) ccw
  arc A99 (4.3256, -0.6029) -> (4.3198, 0.6429) centre (0, 0) ccw
  arc A100 (4.1315, -0.8126) -> (4.3256, -0.6029) centre (4.0779, -0.5684) ccw
  arc A101 (4.0218, -0.8354) -> (4.1315, -0.8126) centre (2.9994, 4.3482) ccw
  arc A102 (3.7602, -0.7206) -> (4.0218, -0.8354) centre (3.9734, -0.5901) ccw
  arc A103 (3.2681, 0.4239) -> (3.7602, -0.7206) centre (7.4854, 1.559) ccw
  arc A104 (2.8013, 0.4197) -> (3.2681, 0.4239) centre (2.9994, 4.3482) ccw
  arc A105 (2.3299, -0.7335) -> (2.8013, 0.4197) centre (-1.4357, 1.4788) ccw
  arc A106 (2.0704, -0.853) -> (2.3299, -0.7335) centre (2.1144, -0.6068) ccw
  arc A107 (1.9603, -0.8321) -> (2.0704, -0.853) centre (2.9994, 4.3482) ccw
  arc A108 (1.7625, -0.6259) -> (1.9603, -0.8321) centre (2.0094, -0.587) ccw
  arc A109 (1.7459, 0.6198) -> (1.7625, -0.6259) centre (6.0765, 0.0546) ccw
  arc A110 (1.3131, 0.7946) -> (1.7459, 0.6198) centre (2.9994, 4.3482) ccw
  arc A111 (0.4362, -0.0904) -> (1.3131, 0.7946) centre (-2.1961, 3.3945) ccw
  arc A112 (0.1507, -0.1015) -> (0.4362, -0.0904) centre (0.2855, 0.109) ccw
  arc A113 (0.057, -0.0401) -> (0.1507, -0.1015) centre (2.9994, 4.3482) ccw
  arc A114 (-0.0469, 0.2261) -> (0.057, -0.0401) centre (0.1962, 0.1676) ccw
  arc A115 (0.4145, 1.3833) -> (-0.0469, 0.2261) centre (4.1992, -0.7961) ccw
  arc A116 (0.0815, 1.7104) -> (0.4145, 1.3833) centre (2.9994, 4.3482) ccw
  arc A117 (-1.0673, 1.2283) -> (0.0815, 1.7104) centre (-2.1656, 5.4553) ccw
  arc A118 (-1.3353, 1.3274) -> (-1.0673, 1.2283) centre (-1.1301, 1.4703) ccw
  arc A119 (-1.3984, 1.42) -> (-1.3353, 1.3274) centre (2.9994, 4.3482) ccw
  arc A120 (-1.3924, 1.7056) -> (-1.3984, 1.42) centre (-1.1903, 1.5586) ccw
  arc A121 (-0.5233, 2.5982) -> (-1.3924, 1.7056) centre (2.1392, -0.8637) ccw
  arc A122 (-0.7058, 3.0279) -> (-0.5233, 2.5982) centre (2.9994, 4.3482) ccw
  arc A123 (-1.9516, 3.0221) -> (-0.7058, 3.0279) centre (-1.3487, 7.3476) ccw
  arc A124 (-2.1613, 3.2161) -> (-1.9516, 3.0221) centre (-1.9171, 3.2697) ccw
  arc A125 (-2.1842, 3.3259) -> (-2.1613, 3.2161) centre (2.9994, 4.3482) ccw
  arc A126 (-2.0694, 3.5875) -> (-2.1842, 3.3259) centre (-1.9389, 3.3742) ccw
  arc A127 (-0.9248, 4.0795) -> (-2.0694, 3.5875) centre (0.2102, -0.1377) ccw
  arc A128 (-0.929, 4.5463) -> (-0.9248, 4.0795) centre (2.9994, 4.3482) ccw
  arc A129 (-2.0822, 5.0177) -> (-0.929, 4.5463) centre (0.1301, 8.7833) ccw
  arc A130 (-2.2017, 5.2772) -> (-2.0822, 5.0177) centre (-1.9556, 5.2333) ccw
  arc A131 (-2.1808, 5.3874) -> (-2.2017, 5.2772) centre (2.9994, 4.3482) ccw
  arc A132 (-1.9747, 5.5851) -> (-2.1808, 5.3874) centre (-1.9357, 5.3382) ccw
  arc A133 (-0.7289, 5.6017) -> (-1.9747, 5.5851) centre (-1.2942, 1.2711) ccw
  arc A134 (-0.5542, 6.0346) -> (-0.7289, 5.6017) centre (2.9994, 4.3482) ccw
  arc A135 (-1.4392, 6.9114) -> (-0.5542, 6.0346) centre (2.0457, 9.5438) ccw
  arc A136 (-1.4503, 7.1969) -> (-1.4392, 6.9114) centre (-1.2397, 7.0621) ccw
  arc A137 (-1.3888, 7.2907) -> (-1.4503, 7.1969) centre (2.9994, 4.3482) ccw
  arc A138 (-1.1227, 7.3945) -> (-1.3888, 7.2907) centre (-1.1812, 7.1514) ccw
  arc A139 (0.0346, 6.9331) -> (-1.1227, 7.3945) centre (-2.1449, 3.1484) ccw
  arc A140 (0.3617, 7.2661) -> (0.0346, 6.9331) centre (2.9994, 4.3482) ccw
  arc A141 (-0.1204, 8.4149) -> (0.3617, 7.2661) centre (4.1066, 9.5132) ccw
  arc A142 (-0.0214, 8.6829) -> (-0.1204, 8.4149) centre (0.1216, 8.4778) ccw
  arc A143 (0.0712, 8.746) -> (-0.0214, 8.6829) centre (2.9994, 4.3482) ccw
  arc A144 (0.3569, 8.7401) -> (0.0712, 8.746) centre (0.2098, 8.5379) ccw
  arc A145 (1.2495, 7.8709) -> (0.3569, 8.7401) centre (-2.2124, 5.2084) ccw
  arc A146 (1.6791, 8.0534) -> (1.2495, 7.8709) centre (2.9994, 4.3482) ccw
  arc A147 (1.6733, 9.2993) -> (1.6791, 8.0534) centre (5.9989, 8.6964) ccw
  arc A148 (1.8674, 9.509) -> (1.6733, 9.2993) centre (1.9209, 9.2648) ccw
  arc A149 (1.9771, 9.5318) -> (1.8674, 9.509) centre (2.9994, 4.3482) ccw
  arc A150 (2.2387, 9.417) -> (1.9771, 9.5318) centre (2.0255, 9.2865) ccw
  arc A151 (2.7308, 8.2725) -> (2.2387, 9.417) centre (-1.4865, 7.1374) ccw
  arc A152 (3.1976, 8.2767) -> (2.7308, 8.2725) centre (2.9994, 4.3482) ccw
  arc A153 (3.669, 9.4299) -> (3.1976, 8.2767) centre (7.4346, 7.2176) ccw
  arc A154 (3.9285, 9.5493) -> (3.669, 9.4299) centre (3.8845, 9.3032) ccw
  arc A155 (4.0386, 9.5285) -> (3.9285, 9.5493) centre (2.9994, 4.3482) ccw
  arc A156 (4.2364, 9.3223) -> (4.0386, 9.5285) centre (3.9894, 9.2833) ccw
  arc A157 (4.253, 8.0766) -> (4.2364, 9.3223) centre (-0.0776, 8.6418) ccw
  arc A158 (4.6858, 7.9018) -> (4.253, 8.0766) centre (2.9994, 4.3482) ccw
  arc A159 (5.5627, 8.7868) -> (4.6858, 7.9018) centre (8.195, 5.3019) ccw
  arc A160 (5.8482, 8.7979) -> (5.5627, 8.7868) centre (5.7134, 8.5873) ccw
  arc A161 (5.9419, 8.7365) -> (5.8482, 8.7979) centre (2.9994, 4.3482) ccw
  arc A162 (6.0457, 8.4703) -> (5.9419, 8.7365) centre (5.8027, 8.5288) ccw
  arc A163 (5.5844, 7.313) -> (6.0457, 8.4703) centre (1.7997, 9.4925) ccw
  arc A164 (5.9174, 6.986) -> (5.5844, 7.313) centre (2.9994, 4.3482) ccw
  arc A165 (7.0662, 7.4681) -> (5.9174, 6.986) centre (8.1645, 3.241) ccw
  arc A166 (7.3341, 7.369) -> (7.0662, 7.4681) centre (7.129, 7.2261) ccw
  arc A167 (7.3973, 7.2764) -> (7.3341, 7.369) centre (2.9994, 4.3482) ccw
  arc A168 (7.3913, 6.9908) -> (7.3973, 7.2764) centre (7.1892, 7.1378) ccw
  arc A169 (6.5222, 6.0982) -> (7.3913, 6.9908) centre (3.8597, 9.5601) ccw
  arc A170 (6.7047, 5.6685) -> (6.5222, 6.0982) centre (2.9994, 4.3482) ccw
  arc A171 (7.9505, 5.6743) -> (6.7047, 5.6685) centre (7.3476, 1.3487) ccw
  arc A172 (8.1602, 5.4803) -> (7.9505, 5.6743) centre (7.916, 5.4267) ccw
  arc A173 (8.1831, 5.3705) -> (8.1602, 5.4803) centre (2.9994, 4.3482) ccw
  arc A174 (8.0683, 5.1089) -> (8.1831, 5.3705) centre (7.9378, 5.3222) ccw
  arc A175 (6.9237, 4.6168) -> (8.0683, 5.1089) centre (5.7887, 8.8341) ccw
  arc A176 (6.9279, 4.1501) -> (6.9237, 4.6168) centre (2.9994, 4.3482) ccw
  arc A177 (8.0811, 3.6787) -> (6.9279, 4.1501) centre (5.8688, -0.0869) ccw
  arc A178 (8.2006, 3.4191) -> (8.0811, 3.6787) centre (7.9545, 3.4631) ccw
  arc A179 (8.1797, 3.309) -> (8.2006, 3.4191) centre (2.9994, 4.3482) ccw
  arc A180 (7.9735, 3.1112) -> (8.1797, 3.309) centre (7.9346, 3.3582) ccw
  arc A181 (6.7278, 3.0946) -> (7.9735, 3.1112) centre (7.2931, 7.4253) ccw
  arc A182 (6.5531, 2.6618) -> (6.7278, 3.0946) centre (2.9994, 4.3482) ccw
  arc A183 (7.4381, 1.7849) -> (6.5531, 2.6618) centre (3.9532, -0.8474) ccw
  arc A184 (7.4491, 1.4995) -> (7.4381, 1.7849) centre (7.2386, 1.6343) ccw
  arc A185 (7.3877, 1.4057) -> (7.4491, 1.4995) centre (2.9994, 4.3482) ccw
  arc A186 (7.1216, 1.3019) -> (7.3877, 1.4057) centre (7.1801, 1.545) ccw
  arc A187 (5.9643, 1.7633) -> (7.1216, 1.3019) centre (8.1438, 5.5479) ccw
  arc A188 (5.6372, 1.4303) -> (5.9643, 1.7633) centre (2.9994, 4.3482) ccw
  arc A189 (6.1193, 0.2815) -> (5.6372, 1.4303) centre (1.8923, -0.8169) ccw
  arc A190 (6.0203, 0.0135) -> (6.1193, 0.2815) centre (5.8773, 0.2186) ccw
  arc A191 (5.9276, -0.0496) -> (6.0203, 0.0135) centre (2.9994, 4.3482) ccw
  arc A192 (5.642, -0.0437) -> (5.9276, -0.0496) centre (5.7891, 0.1585) ccw
  dimension "d64" = 0.05
  constraints: 192 point on circle, 96 centre point, 95 other
  measures "d64" radial gap between concentric circles of A98 A2
extrude "Extrusion11" cut sketch "Sketch13" against normal up to surface (3.25 mm away) contours A95 A94 A93 A92 A91 A90 A89 A88 A87 A86 A85 A84 A83 A82 A81 A80 A79 A78 A77 A76 A75 A74 A73 A72 A71 A70 A69 A68 A67 A66 A65 A64 A63 A62 A61 A60 A59 A58 A57 A56 A55 A54 A53 A52 A51 A50 A49 A48 A47 A46 A45 A44 A43 A42 A41 A40 A39 A38 A37 A36 A35 A34 A33 A32 A31 A30 A29 A28 A27 A26 A25 A24 A23 A22 A21 A20 A19 A18 A17 A16 A15 A14 A13 A12 A11 A10 A9 A8 A7 A6 A5 A4 A3 A2 A1 A0
fillet "Fillet5" radius 0.2 16 edges at (0, -14.45, 4) (7.4782, -14.4433, 4) (19.5, 0, 4) (7.4782, 14.4433, 4) (0, 14.45, 4) (-7.4782, 14.4433, 4) (-19.5, 0, 4) (-7.4782, -14.4433, 4) (-19.5, 0, -4.5) (-7.4782, 14.4433, -4.5) (0, 14.45, -4.5) (7.4782, 14.4433, -4.5) (19.5, 0, -4.5) (7.4782, -14.4433, -4.5) (0, -14.45, -4.5) (-7.4782, -14.4433, -4.5)
body "Solid1"
